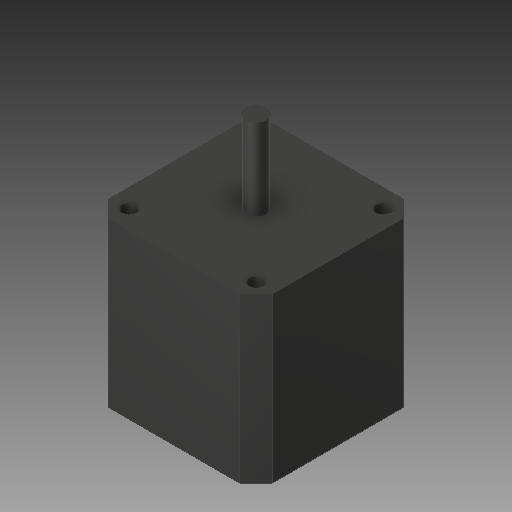
# Autodesk Inventor part: mOTOR
Saved by Autodesk Inventor 2017 (Build 210142000, 142)
## iProperties
Created: 2016-12-11
Part Number: mOTOR
Material: Acetal Resin, Black
Document SubType Name: Modeling
Designer: umr
Density: 1.425 g/cm^3
Appearance: Smooth - Black
Mass: 89.6614 g
Surface Area: 96.9517 cm^2
Volume: 62.9203 cm^3
Author: umr
Autodesk Inventor part; units mm, degrees
ref_plane "YZ Plane" through (0, 0, 0) normal (1, 0, 0) x (0, 1, 0)
ref_plane "XZ Plane" through (0, 0, 0) normal (0, 1, 0) x (-1, 0, 0)
ref_plane "XY Plane" through (0, 0, 0) normal (0, 0, 1) x (1, 0, 0)
sketch "Sketch1" plane through (0, 0, 0) normal (0, 1, 0) x (-1, 0, 0)
  line L0 (0, 0) -> (40, 0)
  line L1 (40, 0) -> (40, -40)
  line L2 (40, -40) -> (0, -40)
  line L3 (0, -40) -> (0, 0)
  dimension "d0" = 40
  dimension "d1" = 40
  constraints: 8 end point, 2 parallel, 1 horizontal, 1 perpendicular
  measures "d0" distance of L1.end L2.end
  measures "d1" distance of L0.end L1.end
extrude "Extrusion1" add sketch "Sketch1" along normal blind 40
chamfer "Chamfer1" distance 4 angle 45 4 edges at (0, 20, 0) (0, 20, -40) (-40, 20, 0) (-40, 20, -40)
sketch "Sketch2" plane through (0, 40, 0) normal (0, 1, 0) x (1, 0, 0)
  circle A0 centre (-20, 20) radius 2.5
  line L0 (-40, 36) -> (-36, 40) projected
  line L1 (-40, 36) -> (-40, 4) projected
  line L2 (-36, 0) -> (-40, 4) projected
  line L3 (-36, 0) -> (-4, 0) projected
  line L4 (0, 4) -> (-4, 0) projected
  line L5 (0, 4) -> (0, 36) projected
  line L6 (-4, 40) -> (0, 36) projected
  line L7 (-4, 40) -> (-36, 40) projected
  point P0 (0, 0)
  dimension "d7" = 5
  dimension "d8" = 40
  dimension "d9" = 20
  dimension "d10" = 20
  constraints: 1 centre point
  measures "d7" diameter of A0
  measures "d8" distance between parallel lines of L3 L7
  measures "d9" horizontal distance of point (0, 0) A0.centre
  measures "d10" distance from line of L5 A0.centre
extrude "Extrusion2" add sketch "Sketch2" along normal blind 20 contours A0
sketch "Sketch3" plane through (0, 40, 0) normal (0, 1, 0) x (1, 0, 0)
  circle A0 centre (-20, 20) radius 2.5 projected
  line L0 (-40, 36) -> (-36, 40) projected
  line L1 (-40, 36) -> (-40, 4) projected
  line L2 (-36, 0) -> (-40, 4) projected
  line L3 (-36, 0) -> (-4, 0) projected
  line L4 (0, 4) -> (-4, 0) projected
  line L5 (0, 4) -> (0, 36) projected
  line L6 (-4, 40) -> (0, 36) projected
  line L7 (-4, 40) -> (-36, 40) projected
  circle A1 centre (-4.5, 4.5) radius 1.75
  circle A2 centre (-4.5, 35.5) radius 1.75
  circle A3 centre (-35.5, 4.5) radius 1.75
  circle A4 centre (-35.5, 35.5) radius 1.75
  point P0 (0, 0)
  dimension "d13" = 3.5
  dimension "d15" = 4
  dimension "d17" = 40
  dimension "d20" = 31
  dimension "d23" = 31
  dimension "d28" = 4.5
  dimension "d29" = 4.5
  constraints: 4 centre point, 1 horizontal, 1 vertical, 6 other
  measures "d13" diameter of A1
  measures "d15" distance of L4.start point (0, 0)
  measures "d17" distance between parallel lines of L7 L3
  measures "d20" distance of A1.centre A2.centre
  measures "d23" distance of A1.centre A3.centre
  measures "d28" distance from line of L5 A1.centre
  measures "d29" distance from line of L3 A3.centre
extrude "Extrusion3" cut sketch "Sketch3" against normal blind 5 contours A1 | A2 | A3 | A4
equation "\"d9\" = 0.5 * d8"
equation "\"d10\" = d9"
equation "\"d28\" = -0.5 * d23 + 0.5 * d17"
equation "\"d29\" = d28"
body "Solid1"
